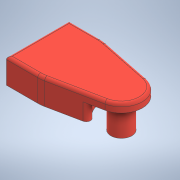
# Autodesk Inventor part: block_01
Saved by Autodesk Inventor 2022 (Build 260153000, 153)
## iProperties
Created: 2022-07-31
Part Number: block_01
Material: Типовые
Document SubType Name: Modeling
Designer: akapu
Density: 1 g/cm^3
Appearance: По умолчанию
Author: akapu
Autodesk Inventor part; units mm, degrees
ref_plane "YZ Plane" through (0, 0, 0) normal (1, 0, 0) x (0, 1, 0)
ref_plane "XZ Plane" through (0, 0, 0) normal (0, 1, 0) x (-1, 0, 0)
ref_plane "XY Plane" through (0, 0, 0) normal (0, 0, 1) x (1, 0, 0)
sketch "Эскиз3" plane through (0, 0, 0) normal (0, 1, 0) x (-1, 0, 0)
  circle A0 centre (0, 0) radius 5.5
  circle A1 centre (0, 0) radius 7.5
  line L0 (7.5, 0) -> (7.5, 7.5)
  line L1 (7.5, 7.5) -> (0, 7.5)
  line L2 (0, 7.5) -> (7.5, 7.5)
  line L3 (7.5, 7.5) -> (7.5, -7.5)
  line L4 (7.5, -7.5) -> (0, -7.5)
  line L5 (0, -7.5) -> (0, 7.5)
  line L6 (-7.5, 0) -> (-12.5, 0)
  circle A2 centre (-12.5, 0) radius 2.5
  circle A3 centre (-12.5, 0) radius 5
  line L7 (-1.5661, -7.3347) -> (-13.4999, -4.899)
  line L8 (-13.5, 4.899) -> (-1.5, 7.3485)
  line L9 (0, 5.5) -> (7.5, 5.5)
  line L10 (0, -5.5) -> (7.5, -5.5)
  line L11 (7.5, -5.5) -> (7.5, -4)
  line L12 (7.5, -4) -> (3.7749, -4)
  line L13 (7.5, 5.5) -> (7.5, 4)
  line L14 (7.5, 4) -> (3.7749, 4)
  circle A4 centre (0, 0) radius 2.45
  dimension "d9" = 11
  dimension "d10" = 15
  dimension "d11" = 5
  dimension "d12" = 5
  dimension "d13" = 1.5
  dimension "d14" = 1.5
  dimension "d17" = 4.9
  constraints: 30 end point, 12 point on circle, 6 perpendicular, 6 point on line, 6 tangent, 5 centre point, 5 coincident, 2 horizontal, 2 parallel, 1 vertical
  measures "d9" diameter of A0
  measures "d10" diameter of A1
  measures "d11" distance of L6.start L6.end
  measures "d12" diameter of A2
  measures "d13" distance of L10.end L11.end
  measures "d14" distance of L9.end L13.end
  measures "d17" diameter of A4
extrude "Выдавливание3" add sketch "Эскиз3" along normal blind 4 contours A0 L14 A1 L12 | A0 L5 A1 | L5 A1 L9 | L14 L0 A1 | L10 A1 L5 | A1 L3 L12 | L1 L0 L9 A1 | A4 L5 | L5 A4 | A1 L10 L3 L4 | A1 A3 L8 | L7 A3 A1 | A2
sketch "Эскиз4" plane through (0, 4, 0) normal (0, 1, 0) x (1, 0, 0)
  circle A0 centre (12.5, 0) radius 2.5 projected
  line L0 (1.5, -7.3485) -> (13.5, -4.899) projected
  circle A1 centre (12.5, 0) radius 5
  line L1 (-7.5, 7.5) -> (-7.5, 5.5) projected
  line L2 (-7.5, -7.5) -> (0, -7.5) projected
  line L3 (-7.5, 7.5) -> (-7.5, -7.5)
  line L4 (-7.5, -7.5) -> (0, -7.5)
  line L5 (1.5, -7.3485) -> (13.5, -4.899)
  arc A2 (1.5661, 7.3347) -> (0, 7.5) centre (0, 0) ccw projected
  line L6 (13.4999, 4.899) -> (1.5661, 7.3347) projected
  line L7 (1.5661, 7.3347) -> (13.4999, 4.899)
  line L8 (-7.5, 7.5) -> (0, 7.5)
  line L9 (0, 7.5) -> (-7.5, 7.5) projected
  circle A3 centre (0, 0) radius 7.5
  point P0 (0, 7.5)
  constraints: 10 end point, 3 collinear, 2 coincident, 1 centre point, 1 perpendicular, 1 point on circle, 1 point on line, 1 tangent, 3 other
extrude "Выдавливание4" add sketch "Эскиз4" along normal blind 2 contours A0 | A3 A1 L0 | A3 A2 | A1 | L2 L3 A3 | A3 L6 A1 | L3 L1 L8 A3
fillet "Сопряжение1" radius 1 2 edges at (13.5, 2, 4.899) (13.4999, 2, -4.899)
sketch "Эскиз5" plane through (0, 0, 0) normal (0, -1, 0) x (1, 0, 0)
  circle A0 centre (0, 0) radius 2.475
  circle A1 centre (12.5, 0) radius 2.5 projected
  circle A2 centre (12.5, 0) radius 2.5
  dimension "d25" = 4.95
  constraints: 2 centre point, 2 coincident
  measures "d25" diameter of A0
extrude "Выдавливание5" add sketch "Эскиз5" along normal blind 3 and the other way blind 5
fillet "Сопряжение3" radius 0.7 16 edges at (17.5, 6, -0.0001) (7.533, 6, -6.1168) (0.7538, 6, 7.462) (-3.75, 6, 7.5) (7.5, 6, 6.1237) (-7.5, 6, 0) (0.7874, 6, -7.4586) (-3.75, 6, -7.5) (-3.7749, 2, 4) (-3.7749, 2, -4) (-7.5, 2, -4) (-7.5, 2, -5.5) (-7.5, 4, -4.75) (-7.5, 2, 5.5) (-7.5, 2, 4) (-7.5, 4, 4.75)
